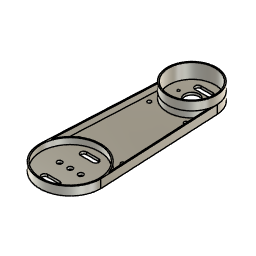
TRARM02_Link3A_100x50x7 (Autodesk Fusion 360 design; units mm, degrees)
Autodesk Fusion 360 part; units mm, degrees
sketch "스케치1" plane through (0, 0, 0) normal (0, 0, 1) x (1, 0, 0)
  line L0 (19.9753, 100.9938) -> (25, 0)
  line L1 (-19.9753, 100.9938) -> (-25, 0)
  arc A0 (19.9753, 100.9938) -> (-19.9753, 100.9938) centre (0, 100) ccw
  arc A1 (-25, 0) -> (25, 0) centre (0, 0) ccw
  dimension "d1" = 50
  dimension "d222" = 20
  dimension "d223" = 100
  constraint coincident A1.centre origin
  constraint tangent L1 A0
  constraint horizontal A1.centre L1.end
  constraint horizontal A1.centre L0.end
  constraint vertical A1.centre A0.centre
  constraint tangent L0 A0
  measures "d1" diameter of A1
  measures "d222" radius of A0
  measures "d223" distance of A1.centre A0.centre
extrude "돌출1" add sketch "스케치1" along normal blind 2
sketch "스케치2" plane through (0, 0, 2) normal (0, 0, 1) x (-1, 0, 0)
  arc A0 (-19.9753, -100.9938) -> (19.9753, -100.9938) centre (0, -100) ccw
  line L0 (19.9753, -100.9938) -> (25, 0)
  line L1 (-25, 0) -> (-19.9753, -100.9938)
  line L2 (19.9753, -100.9938) -> (25, 0)
  arc A1 (-19.9753, -100.9938) -> (19.9753, -100.9938) centre (0, -100) ccw
  line L3 (-25, 0) -> (-19.9753, -100.9938)
  arc A2 (25, 0) -> (-25, 0) centre (0, 0) ccw
  line L4 (-23.5864, -8.2873) -> (-19.2868, -94.7068)
  line L5 (19.2868, -94.7068) -> (23.5864, -8.2873)
  circle A3 centre (0, -100) radius 19
  circle A4 centre (0, 0) radius 23.9691
  arc A5 (-23.5864, -8.2873) -> (23.5864, -8.2873) centre (0, 0) ccw
  arc A6 (25, 0) -> (-25, 0) centre (0, 0) ccw
  arc A7 (-19.9753, -100.9938) -> (19.9753, -100.9938) centre (0, -100) ccw
  arc A8 (19.2868, -94.7068) -> (-19.2868, -94.7068) centre (0, -100) ccw
  constraint concentric A0 A7
  constraint concentric A1 A3
  constraint tangent L4 A3
  constraint concentric A2 A5
  constraint coincident L1.start A5
  constraint concentric A2 A4
  constraint tangent L4 A4
  constraint concentric A5 A6
  constraint coincident L5.start A7
  constraint concentric A7 A8
extrude "돌출25" add sketch "스케치2" along normal blind 5
sketch "스케치22" plane through (0, 0, 2) normal (0, 0, 1) x (-1, 0, 0)
  circle A0 centre (0, 0) radius 2
  circle A1 centre (-8.7, 0) radius 2
  circle A2 centre (8.7, 0) radius 2
  circle A3 centre (0, -100) radius 6
  circle A4 centre (-11, -100) radius 1
  circle A5 centre (11, -100) radius 1
  dimension "d208" = 4
  dimension "d209" = 8.7
  dimension "d210" = 8.7
  dimension "d226" = 12
  dimension "d227" = 2
  dimension "d228" = 11
  dimension "d229" = 11
  dimension "d230" = 100
  constraint coincident A0.centre origin
  constraint equal A0 A2
  constraint equal A0 A1
  constraint horizontal A0.centre A1.centre
  constraint horizontal A0.centre A2.centre
  constraint equal A4 A5
  constraint horizontal A3.centre A5.centre
  constraint horizontal A3.centre A4.centre
  constraint vertical A0.centre A3.centre
  measures "d208" diameter of A0
  measures "d209" distance of A0.centre A1.centre
  measures "d210" distance of A0.centre A2.centre
  measures "d226" diameter of A3
  measures "d227" diameter of A4
  measures "d228" distance of A3.centre A4.centre
  measures "d229" distance of A3.centre A5.centre
  measures "d230" distance of A0.centre A3.centre
extrude "돌출26" cut sketch "스케치22" against normal blind 2
sketch "스케치24" plane through (0, 0, 7) normal (0, 0, 1) x (-1, 0, 0)
  circle A0 centre (0, -100) radius 20
  circle A1 centre (0, -100) radius 6
  arc A2 (-19.9753, -100.9938) -> (19.9753, -100.9938) centre (0, -100) ccw
  circle A3 centre (0, -100) radius 19
  circle A4 centre (0, -100) radius 19
  constraint concentric A0 A1
  constraint tangent A0 A2
  constraint concentric A1 A3
  constraint tangent A3 A4
extrude "돌출28" add sketch "스케치24" along normal blind 7 contours A0 A2
sketch "스케치23" plane through (0, 0, 2) normal (0, 0, 1) x (-1, 0, 0)
  circle A0 centre (-18, -25) radius 1.5
  circle A1 centre (-15, -80) radius 1.5
  circle A2 centre (15, -80) radius 1.5
  circle A3 centre (18, -25) radius 1.5
  circle A4 centre (0, -100) radius 6
  dimension "d214" = 3
  dimension "d215" = 18
  dimension "d216" = 18
  dimension "d217" = 25
  dimension "d225" = 20
  dimension "d233" = 15
  dimension "d234" = 15
  constraint equal A0 A3
  constraint equal A0 A1
  constraint equal A1 A2
  constraint horizontal A1.centre A2.centre
  constraint horizontal A0.centre A3.centre
  measures "d214" diameter of A0
  measures "d215" horizontal distance of origin A0.centre
  measures "d216" horizontal distance of origin A3.centre
  measures "d217" vertical distance of origin A0.centre
  measures "d225" vertical distance of A1.centre A4.centre
  measures "d233" horizontal distance of A1.centre A4.centre
  measures "d234" horizontal distance of A2.centre A4.centre
extrude "돌출27" cut sketch "스케치23" against normal blind 2 contours A0 | A1 | A2 | A3
sketch "스케치26" plane through (0, 0, 2) normal (0, 0, 1) x (-1, 0, 0)
  line L0 (5, -13.5) -> (-5, -13.5)
  line L1 (5, -18.5) -> (-5, -18.5)
  arc A0 (-5, -13.5) -> (-5, -18.5) centre (-5, -16) ccw
  arc A1 (5, -18.5) -> (5, -13.5) centre (5, -16) ccw
  line L2 (5, 13.5) -> (-5, 13.5)
  line L3 (5, 18.5) -> (-5, 18.5)
  arc A2 (5, 13.5) -> (5, 18.5) centre (5, 16) ccw
  arc A3 (-5, 18.5) -> (-5, 13.5) centre (-5, 16) ccw
  line L4 (5, -112.5) -> (-5, -112.5)
  line L5 (5, -107.5) -> (-5, -107.5)
  arc A4 (5, -112.5) -> (5, -107.5) centre (5, -110) ccw
  arc A5 (-5, -107.5) -> (-5, -112.5) centre (-5, -110) ccw
  line L6 (4.5597, -92.4609) -> (-4.9898, -92.5)
  line L7 (5, -87.5) -> (-5, -87.5)
  arc A6 (4.5597, -92.4609) -> (5, -87.5) centre (5, -90) ccw
  arc A7 (-5, -87.5) -> (-4.9898, -92.5) centre (-5, -90) ccw
  circle A8 centre (0, -100) radius 6
  dimension "d235" = 5
  dimension "d236" = 10
  dimension "d239" = 16
  dimension "d241" = 5
  dimension "d242" = 5
  dimension "d243" = 10
  dimension "d244" = 16
  dimension "d245" = 5
  dimension "d248" = 5
  dimension "d249" = 10
  dimension "d250" = 10
  dimension "d251" = 10
  dimension "d252" = 5
  constraint equal A0 A1
  constraint horizontal A0.centre A1.centre
  constraint horizontal L0
  constraint horizontal L1
  constraint tangent L1 A0
  constraint tangent L0 A0
  constraint equal A2 A3
  constraint tangent L2 A3
  constraint horizontal L2
  constraint tangent L3 A3
  constraint parallel L2 L3
  constraint equal A6 A7
  constraint equal A5 A7
  constraint equal A4 A5
  constraint vertical A4.centre A6.centre
  constraint vertical A5.centre A7.centre
  constraint horizontal A5.centre A4.centre
  constraint horizontal L4
  constraint horizontal L5
  constraint tangent L4 A5
  constraint tangent L5 A5
  constraint horizontal A7.centre A6.centre
  constraint horizontal L7
  constraint tangent L6 A7
  constraint tangent L7 A7
  measures "d235" diameter of A0
  measures "d236" distance of A0.centre A1.centre
  measures "d239" vertical distance of origin A0.centre
  measures "d241" horizontal distance of origin L0.end
  measures "d242" diameter of A3
  measures "d243" distance of A2.centre A3.centre
  measures "d244" vertical distance of origin A3.centre
  measures "d245" horizontal distance of origin A3.centre
  measures "d248" diameter of A5
  measures "d249" distance of A5.centre A4.centre
  measures "d250" vertical distance of A5.centre A8.centre
  measures "d251" vertical distance of A7.centre A8.centre
  measures "d252" horizontal distance of A7.centre A8.centre
extrude "돌출29" cut sketch "스케치26" against normal blind 2 contours L0 L1 A0 A1 | L2 L3 A2 A3 | L4 L5 A4 A5 | L6 L7 A6 A7
